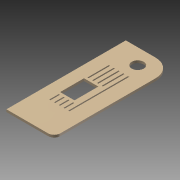
# Autodesk Inventor part: base_lateral_cover_rigth_v2
Saved by Autodesk Inventor 2015 (Build 190159000, 159)
## iProperties
Created: 2016-05-01
Part Number: base_lateral_cover_rigth_v2
Material: Plástico ABS
Document SubType Name: Modeling
Designer: JavierPC
Density: 1.06 g/cm^3
Appearance: Suave - Color hueso
Author: Javier Pérez de Frutos
Title: Lateral del módulo central
Autodesk Inventor part; units mm, degrees
ref_plane "YZ Plane" through (0, 0, 0) normal (1, 0, 0) x (0, 1, 0)
ref_plane "XZ Plane" through (0, 0, 0) normal (0, 1, 0) x (-1, 0, 0)
ref_plane "XY Plane" through (0, 0, 0) normal (0, 0, 1) x (1, 0, 0)
sketch "Boceto1" plane through (0, 0, 0) normal (0, 0, 1) x (1, 0, 0)
  line L0 (-20, 50) -> (5, 50)
  line L1 (20, 35) -> (20, -45)
  line L2 (15, -50) -> (-20, -50)
  line L3 (-20, -50) -> (-20, 50)
  line L4 (0, 26.3033) -> (0, -44.8052)
  line L5 (-41.9778, 0) -> (28.2031, 0)
  arc A0 (20, 35) -> (5, 50) centre (5, 35) ccw
  arc A1 (15, -50) -> (20, -45) centre (15, -45) ccw
  point P0 (0, 0)
  point P1 (0, 50)
  point P2 (-20, 0)
  dimension "d3" = 30
  dimension "d4" = 10
  dimension "d5" = 100
  dimension "d6" = 40
  constraints: 12 end point, 4 point on circle, 4 tangent, 3 horizontal, 3 point on line, 2 centre point, 2 parallel, 2 vertical, 1 midpoint, 1 perpendicular
  measures "d3" diameter of A0
  measures "d4" diameter of A1
  measures "d5" diameter of L0 L5
  measures "d6" diameter of L3 L4
extrude "Extrusión1" add sketch "Boceto1" along normal blind 2
sketch "Boceto2" plane through (0, 0, 2) normal (0, 0, 1) x (1, 0, 0)
  line L0 (-20, -50) -> (15, -50) projected
  line L1 (20, -45) -> (20, 35) projected
  line L2 (5, 50) -> (-20, 50) projected
  line L3 (-20, 50) -> (-20, -50) projected
  circle A0 centre (-10, 47.5) radius 1
  circle A1 centre (17.5, 35) radius 1
  circle A2 centre (17.5, 15) radius 1
  circle A3 centre (17.5, -5) radius 1
  circle A4 centre (17.5, -25) radius 1
  circle A5 centre (17.5, -45) radius 1
  circle A6 centre (-15, -47.5) radius 1
  point P0 (0, 0)
  dimension "d9" = 2.5
  dimension "d10" = 5
  dimension "d11" = 5
  dimension "d12" = 2.5
  dimension "d13" = 2.5
  dimension "d14" = 2.5
  dimension "d15" = 2.5
  dimension "d16" = 2.5
  dimension "d17" = 10
  dimension "d18" = 20
  dimension "d19" = 20
  dimension "d20" = 20
  dimension "d21" = 2.5
  dimension "d22" = 20
  dimension "d23" = 2
  dimension "d24" = 2
  dimension "d25" = 2
  dimension "d26" = 2
  dimension "d27" = 2
  dimension "d28" = 2
  dimension "d29" = 2
  constraints: 7 centre point, 7 coincident
  measures "d9" distance from line of L0 point (-15, -47.5)
  measures "d10" horizontal distance of point (-15, -47.5) L0.start
  measures "d11" distance from line of L0 point (17.5, -45)
  measures "d12" distance from line of L1 point (17.5, -45)
  measures "d13" distance from line of L1 point (17.5, -25)
  measures "d14" distance from line of L1 point (17.5, -5)
  measures "d15" distance from line of L1 point (17.5, 15)
  measures "d16" distance from line of L2 point (-10, 47.5)
  measures "d17" distance from line of L3 point (-10, 47.5)
  measures "d18" distance of point (17.5, -45) point (17.5, -25)
  measures "d19" distance of point (17.5, -5) point (17.5, -25)
  measures "d20" distance of point (17.5, 15) point (17.5, -5)
  measures "d21" distance from line of L1 point (17.5, 35)
  measures "d22" distance of point (17.5, 15) point (17.5, 35)
  measures "d23" diameter of A0
  measures "d24" diameter of A1
  measures "d25" diameter of A2
  measures "d26" diameter of A3
  measures "d27" diameter of A4
  measures "d28" diameter of A5
  measures "d29" diameter of A6
extrude "Extrusión2" [suppressed]
sketch "Boceto3" plane through (0, 0, 0) normal (0, 0, -1) x (-1, 0, 0)
  line L0 (20, -50) -> (20, 50) projected
  line L1 (20, 50) -> (-5, 50) projected
  point P0 (0, 0)
  point P1 (-3, 37)
  dimension "d32" = 23
  dimension "d33" = 13
  measures "d32" distance from line of L0 point (-3, 37)
  measures "d33" distance from line of L1 point (-3, 37)
hole "Agujero1" at (3, 37, 0) direction (0, 0, 1) diameter 10 end through all
sketch "Boceto4" plane through (0, 0, 0) normal (0, 0, 1) x (1, 0, 0)
  line L0 (-8.1395, 25) -> (-9.1395, 25)
  line L1 (-9.1395, 25) -> (-9.1395, -25)
  line L2 (-9.1395, -25) -> (-8.1395, -25)
  line L3 (-8.1395, -25) -> (-8.1395, 25)
  line L4 (-48.3206, 0) -> (41.5333, 0)
  line L5 (-4.1395, 25) -> (-5.1395, 25)
  line L6 (-5.1395, 25) -> (-5.1395, -25)
  line L7 (-5.1395, -25) -> (-4.1395, -25)
  line L8 (-4.1395, -25) -> (-4.1395, 25)
  line L9 (-0.1395, 25) -> (-1.1395, 25)
  line L10 (-1.1395, 25) -> (-1.1395, -25)
  line L11 (-1.1395, -25) -> (-0.1395, -25)
  line L12 (-0.1395, -25) -> (-0.1395, 25)
  line L13 (3.8605, 25) -> (2.8605, 25)
  line L14 (2.8605, 25) -> (2.8605, -25)
  line L15 (2.8605, -25) -> (3.8605, -25)
  line L16 (3.8605, -25) -> (3.8605, 25)
  line L17 (7.8605, 25) -> (6.8605, 25)
  line L18 (6.8605, 25) -> (6.8605, -25)
  line L19 (6.8605, -25) -> (7.8605, -25)
  line L20 (7.8605, -25) -> (7.8605, 25)
  point P0 (0, 0)
  point P1 (-9.1395, 0)
  dimension "d41" = 1
  dimension "d42" = 50
  dimension "d43" = 1
  dimension "d44" = 50
  dimension "d45" = 1
  dimension "d46" = 50
  dimension "d47" = 1
  dimension "d48" = 50
  dimension "d49" = 1
  dimension "d50" = 50
  dimension "d51" = 3
  dimension "d52" = 3
  dimension "d53" = 3
  dimension "d54" = 3
  constraints: 42 end point, 10 parallel, 7 horizontal, 5 perpendicular, 1 midpoint, 1 point on line
  measures "d41" distance of L2.end L1.end
  measures "d42" distance of L1.end L0.end
  measures "d43" distance of L7.end L6.end
  measures "d44" distance of L6.end L5.end
  measures "d45" distance of L11.end L10.end
  measures "d46" distance of L10.end L9.end
  measures "d47" distance of L15.end L14.end
  measures "d48" distance of L14.end L13.end
  measures "d49" distance of L19.end L18.end
  measures "d50" distance of L18.end L17.end
  measures "d51" distance between parallel lines of L3 L6
  measures "d52" distance between parallel lines of L10 L8
  measures "d53" distance between parallel lines of L14 L12
  measures "d54" distance between parallel lines of L18 L16
extrude "Extrusión3" cut sketch "Boceto4" along normal blind 10
sketch "Boceto5" plane through (0, 0, 0) normal (0, 0, 1) x (1, 0, 0)
  line L0 (5, 50) -> (-20, 50) projected
  line L1 (20, -45) -> (20, 35) projected
  line L2 (-20, -50) -> (-20, 50) projected
  line L3 (2, 63.3665) -> (2, 50)
  line L4 (2, 5) -> (2, -15)
  line L5 (-10, 55.864) -> (-10, 50)
  line L6 (-10, 5) -> (-10, -15)
  line L7 (-56.3903, 5) -> (-20, 5)
  line L8 (-10, 5) -> (2, 5)
  line L9 (20, 5) -> (36.1498, 5)
  line L10 (20, -15) -> (39.7486, -15)
  line L11 (-56.3903, -15) -> (-20, -15)
  line L12 (-10, -15) -> (2, -15)
  point P0 (0, 0)
  dimension "d61" = 10
  dimension "d62" = 20
  dimension "d63" = 45
  dimension "d64" = 12
  constraints: 20 end point, 6 horizontal, 6 point on line, 4 vertical
  measures "d61" distance between parallel lines of L2 L6
  measures "d62" distance between parallel lines of L8 L12
  measures "d63" distance between parallel lines of L0 L8
  measures "d64" distance between parallel lines of L6 L4
extrude "Extrusión4" cut sketch "Boceto5" along normal blind 10
sketch "Boceto6" plane through (0, 0, 0) normal (0, 0, 1) x (1, 0, 0)
  line L0 (-10, -15) -> (2, -15)
  line L1 (2, -15) -> (2, 5)
  line L2 (2, 5) -> (-10, 5)
  line L3 (-10, 5) -> (-10, -15)
  line L4 (-12, -17) -> (4, -17)
  line L5 (4, -17) -> (4, 7)
  line L6 (4, 7) -> (-12, 7)
  line L7 (-12, 7) -> (-12, -17)
  point P0 (0, 0)
  point P1 (2, -15)
  point P2 (-10, 5)
  dimension "d67" = 2
  constraints: 16 end point, 4 parallel, 2 perpendicular, 1 horizontal, 3 other
  measures "d67" distance between parallel lines of L3 L7
extrude "Extrusión5" add sketch "Boceto6" along normal up to surface (2 mm away)
